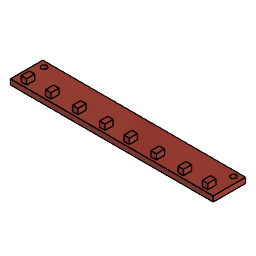
line_sensor (Autodesk Fusion 360 design; units mm, degrees)
part number: 2025-11-20-19-18-52-601
Autodesk Fusion 360 part; units mm, degrees
sketch "Szkic1" plane through (0, 0, 0) normal (0, 0, 1) x (1, 0, 0)
  line L0 (0, 0) -> (75, 0)
  line L1 (75, 0) -> (75, 12)
  line L2 (75, 12) -> (0, 12)
  line L3 (0, 12) -> (0, 0)
  dimension "d1" = 75
  dimension "d2" = 12
  constraint horizontal L0
  constraint vertical L1
  constraint horizontal L2
  constraint vertical L3
  constraint coincident L0.start L3.end
  measures "d1" distance of L0.start L0.end
  measures "d2" distance of L0.start L2.end
extrude "Wyciągnięcie proste1" add sketch "Szkic1" along normal blind 2
sketch "Szkic2" plane through (0, 0, 2) normal (0, 0, 1) x (-1, 0, 0)
  line L0 (0, -12) -> (0, 0)
  line L1 (0, 0) -> (-75, 0)
  line L2 (-75, 0) -> (-75, -12)
  line L3 (-75, -12) -> (0, -12)
  line L4 (-3, -1) -> (-5, -1)
  line L5 (-5, -1) -> (-5, -4)
  line L6 (-5, -4) -> (-3, -4)
  line L7 (-3, -4) -> (-3, -1)
  line L8 (-72, -1) -> (-70, -1)
  line L9 (-70, -1) -> (-70, -4)
  line L10 (-70, -4) -> (-72, -4)
  line L11 (-72, -4) -> (-72, -1)
  line L12 (-12, -1) -> (-14, -1)
  line L13 (-14, -1) -> (-14, -4)
  line L14 (-14, -4) -> (-12, -4)
  line L15 (-12, -4) -> (-12, -1)
  line L16 (-63, -1) -> (-61, -1)
  line L17 (-61, -1) -> (-61, -4)
  line L18 (-61, -4) -> (-63, -4)
  line L19 (-63, -4) -> (-63, -1)
  line L20 (-22, -1) -> (-24, -1)
  line L21 (-24, -1) -> (-24, -4)
  line L22 (-24, -4) -> (-22, -4)
  line L23 (-22, -4) -> (-22, -1)
  line L24 (-53, -1) -> (-51, -1)
  line L25 (-51, -1) -> (-51, -4)
  line L26 (-51, -4) -> (-53, -4)
  line L27 (-53, -4) -> (-53, -1)
  line L28 (-32, -1) -> (-34, -1)
  line L29 (-34, -1) -> (-34, -4)
  line L30 (-34, -4) -> (-32, -4)
  line L31 (-32, -4) -> (-32, -1)
  line L32 (-43, -1) -> (-41, -1)
  line L33 (-41, -1) -> (-41, -4)
  line L34 (-41, -4) -> (-43, -4)
  line L35 (-43, -4) -> (-43, -1)
  constraint horizontal L4
  constraint vertical L5
  constraint horizontal L6
  constraint vertical L7
  constraint horizontal L8
  constraint vertical L9
  constraint horizontal L10
  constraint vertical L11
  constraint horizontal L12
  constraint vertical L13
  constraint horizontal L14
  constraint vertical L15
  constraint horizontal L16
  constraint vertical L17
  constraint horizontal L18
  constraint vertical L19
  constraint horizontal L20
  constraint vertical L21
  constraint horizontal L22
  constraint vertical L23
  constraint horizontal L24
  constraint vertical L25
  constraint horizontal L26
  constraint vertical L27
  constraint horizontal L28
  constraint vertical L29
  constraint horizontal L30
  constraint vertical L31
  constraint horizontal L32
  constraint vertical L33
  constraint horizontal L34
  constraint vertical L35
extrude "Wyciągnięcie proste2" add sketch "Szkic2" along normal blind 2 contours L4 L5 L6 L7 | L8 L9 L10 L11 | L12 L13 L14 L15 | L16 L17 L18 L19 | L20 L21 L22 L23 | L24 L25 L26 L27 | L28 L29 L30 L31 | L32 L33 L34 L35
sketch "Szkic3" plane through (0, 0, 0) normal (0, 0, -1) x (1, 0, 0)
  line L0 (0, 0) -> (0, -12)
  line L1 (0, -12) -> (75, -12)
  line L2 (75, -12) -> (75, 0)
  line L3 (75, 0) -> (0, 0)
  circle A0 centre (2.5, -10) radius 1
  circle A1 centre (72.5, -10) radius 1
  dimension "d8" = 2
  dimension "d9" = 2
  measures "d8" diameter of A0
  measures "d9" diameter of A1
extrude "Wyciągnięcie proste3" cut sketch "Szkic3" against normal blind 4 contours A0 | A1
named bodies: "czujnik"
